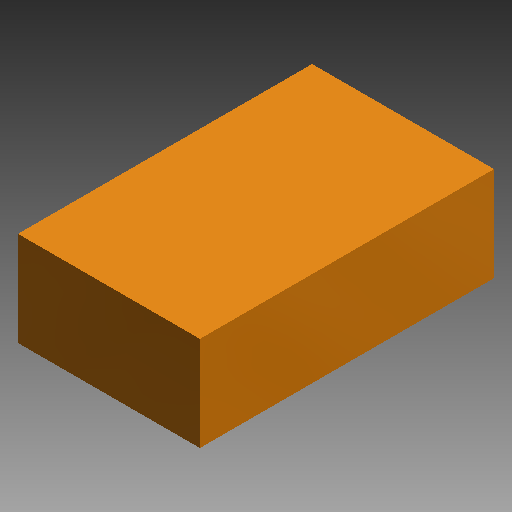
# Autodesk Inventor part: M02PTH
Saved by Autodesk Inventor 2018.2 (Build 222227000, 227)
## iProperties
Part Number: M02PTH
Material: Generic
Document SubType Name: Modeling
Designer: autocad
Appearance: 1X02, M02PTH
Author: autocad
Autodesk Inventor part; units mm, degrees
ref_plane "YZ Plane" through (0, 0, 0) normal (1, 0, 0) x (0, 1, 0)
ref_plane "XZ Plane" through (0, 0, 0) normal (0, 1, 0) x (-1, 0, 0)
ref_plane "XY Plane" through (0, 0, 0) normal (0, 0, 1) x (1, 0, 0)
sketch "1X02, M02PTH_177" plane through (0, 0, 0) normal (0, 0, 1) x (1, 0, 0)
  line L0 (3.9116, -1.3716) -> (-1.3716, -1.3716)
  line L1 (-1.3716, -1.3716) -> (-1.3716, 1.3716)
  line L2 (-1.3716, 1.3716) -> (3.9116, 1.3716)
  line L3 (3.9116, 1.3716) -> (3.9116, -1.3716)
  constraints: 8 end point
extrude "Extrusion1" add sketch "1X02, M02PTH_177" along normal blind 8.54
body "Solid1"
